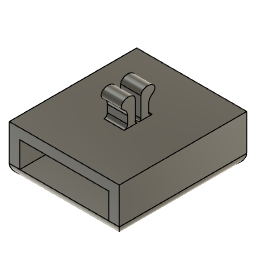
ender5-sd-card-adapter (Autodesk Fusion 360 design; units mm, degrees)
Autodesk Fusion 360 part; units mm, degrees
sketch "Sketch2" plane through (0, 0, 0) normal (0, 0, 1) x (1, 0, 0)
  line L0 (-4.2973, 17.5066) -> (3.1027, 17.5066)
  line L1 (3.1027, 17.5066) -> (3.1027, -15.9934)
  line L2 (3.1027, -15.9934) -> (-4.2973, -15.9934)
  line L3 (-4.2973, -15.9934) -> (-4.2973, 17.5066)
  dimension "d9" = 7.4
  dimension "d10" = 33.5
  constraint horizontal L0
  constraint vertical L1
  constraint horizontal L2
  constraint vertical L3
  measures "d9" distance of L0.start L0.end
  measures "d10" distance of L0.start L2.end
extrude "Extrude1" add sketch "Sketch2" along normal blind 25.5 makes body 1
shell "Shell1" thickness 3 outward yes removed faces 1 at (0.636, -15.9934, 8.5) on bodies 1
sketch "Sketch5" plane through (6.1027, 0, 0) normal (1, 0, 0) x (0, 1, 0)
  line L0 (-15.9934, -3) -> (20.5066, -3)
  line L1 (20.5066, -3) -> (20.5066, 28.5)
  line L2 (20.5066, 28.5) -> (-15.9934, 28.5)
  line L3 (-15.9934, 28.5) -> (-15.9934, -3)
  line L4 (2.2566, 28.5) -> (2.2566, -3) construction
  line L5 (-15.9934, 12.75) -> (20.5066, 12.75) construction
  line L6 (-0.7434, 15.65) -> (1.4566, 15.65)
  line L7 (1.4566, 15.65) -> (1.4566, 9.85)
  line L8 (1.4566, 9.85) -> (-0.7434, 9.85)
  line L9 (-0.7434, 9.85) -> (-0.7434, 15.65)
  line L10 (5.2566, 9.85) -> (5.2566, 15.65)
  line L11 (5.2566, 15.65) -> (3.0566, 15.65)
  line L12 (3.0566, 15.65) -> (3.0566, 9.85)
  line L13 (3.0566, 9.85) -> (5.2566, 9.85)
  dimension "d30" = 5.8
  dimension "d31" = 3
  dimension "d32" = 2.2
  dimension "d33" = 2.9
  constraint midpoint L2 L4.start
  constraint midpoint L0 L4.end
  constraint midpoint L3 L5.start
  constraint midpoint L1 L5.end
  constraint horizontal L6
  constraint vertical L7
  constraint horizontal L8
  constraint vertical L9
  constraint symmetric L4 L6.start L10.end
  constraint symmetric L4 L6.end L11.end
  constraint symmetric L4 L7.end L12.end
  constraint symmetric L4 L8.end L10.start
  measures "d30" distance of L6.start L8.end
  measures "d31" distance of L4 L9
  measures "d32" distance of L6.start L6.end
  measures "d33" distance of L5 L6
extrude "Extrude5" add sketch "Sketch5" along normal blind 6.2 contours L6 L7 L8 L9 | L10 L11 L12 L13 bodies 1
sketch "Sketch7" plane through (0, 0, 15.65) normal (0, 0, 1) x (-1, 0, 0)
  line L0 (-6.1027, -1.4566) -> (-6.1027, 0.7434)
  line L1 (-6.1027, 0.7434) -> (-12.3027, 0.7434)
  line L2 (-12.3027, 0.7434) -> (-12.3027, -1.4566)
  line L3 (-12.3027, -1.4566) -> (-6.1027, -1.4566)
  ellipse E0 centre (-12.3027, 0.5434) end of major axis (-13.8027, 0.5434) minor radius 2
  line L4 (-10.8027, 0.5434) -> (-13.8027, 0.5434)
  line L5 (-12.3027, 2.5434) -> (-12.3027, -1.4566)
  dimension "d41" = 3
  dimension "d42" = 4
  constraint perpendicular L2 L4
  constraint coincident E0 L4.start
  constraint coincident E0 L4.end
  constraint coincident E0 L5.start
  constraint coincident E0 L2.end
  constraint coincident L2.end L3.start
  measures "d41" distance of E0
extrude "Extrude7" add sketch "Sketch7" against normal blind 5.8 contours L2 E0 L4 L5 | L2 E0 L4 L5 | L1 L2 E0 L4 L5 | L1 E0 L5 | L2 E0 L4 L5 bodies 1
fillet "Fillet1" radius 2.25 1 edges at (10.8102, -0.7434, 12.75) on bodies 1
ref_plane "WorkPlane2" through (9.2027, 2.2566, 12.75) normal (0, 1, 0) x (0, 0, 1)
mirror "Mirror2" about plane through (9.2027, 2.2566, 12.75) normal (0, 1, 0) of "Extrude7", "Fillet1"
sketch "Sketch8" plane through (0, 0, 15.65) normal (0, 0, 1) x (-1, 0, 0)
  line L0 (-6.1027, -5.2566) -> (-6.1027, -3.0566)
  line L1 (-6.1027, -3.0566) -> (-12.3027, -3.0566)
  ellipse E0 centre (-12.3027, -5.0566) end of major axis (-12.3027, -3.0566) minor radius 1.5 (-12.3027, -3.0566) -> (-11.1437, -6.3262) ccw
  arc A0 (-9.2282, -5.2566) -> (-11.1437, -6.3262) centre (-9.2282, -7.5066) ccw
  line L2 (-9.2282, -5.2566) -> (-6.1027, -5.2566)
fillet "Fillet2" radius 0.55 2 edges at (6.1027, 3.0566, 12.75) (6.1027, 1.4566, 12.75) on bodies 1
sketch "Sketch1" plane through (0, 0, 0) normal (1, 0, 0) x (0, 1, 0) in component "SDCardThing"
  line L0 (-16.5, -12.5) -> (16.5, -12.5)
  line L1 (16.5, -12.5) -> (16.5, 12.5)
  line L2 (16.5, 12.5) -> (-16.5, 12.5)
  line L3 (-16.5, 12.5) -> (-16.5, -12.5)
  line L4 (-16.5, -12.5) -> (16.5, 12.5) construction
  line L5 (16.5, -12.5) -> (-16.5, 12.5) construction
  dimension "d48" = 33
  dimension "d49" = 25
  constraint horizontal L0
  constraint perpendicular L0 L1
  constraint parallel L0 L2
  constraint parallel L1 L3
  constraint coincident L4 origin
  constraint coincident L5 origin
  measures "d48" distance of L1.end L2.end
  measures "d49" distance of L0.end L1.end
extrude "Extrude1'" add sketch "Sketch1" along normal blind 7.2 separate body makes body 2 in component "SDCardThing"
move_body "Move1" bodies 2 to x (1, 0, 0) y (0, 1, 0) z (0, 0, 1) at (1, 3, 0) in component "SDCardThing"
sketch "Sketch2 (2)" plane through (0, 19.5, 0) normal (0, 1, 0) x (-1, 0, 0) in component "SDCardThing"
  line L0 (-1, -12.5) -> (-1, 12.5)
  line L1 (-1, 12.5) -> (-8.2, 12.5)
  line L2 (-8.2, 12.5) -> (-8.2, -12.5)
  line L3 (-8.2, -12.5) -> (-1, -12.5)
  line L4 (-5.1, -5.5) -> (-4.1, -5.5)
  line L5 (-4.1, -5.5) -> (-4.1, 5.5)
  line L6 (-4.1, 5.5) -> (-5.1, 5.5)
  line L7 (-5.1, 5.5) -> (-5.1, -5.5)
  point P0 (-5.1, 0)
  point P1 (-8.2, 0)
  point P2 (-4.6, -5.5)
  point P3 (-4.6, -12.5)
  dimension "d53" = 1
  dimension "d54" = 11
  constraint horizontal L4
  constraint vertical L5
  constraint horizontal L6
  constraint vertical L7
  constraint midpoint L7 P0
  constraint midpoint L2 P1
  constraint horizontal P0 P1
  constraint midpoint L4 P2
  constraint midpoint L3 P3
  constraint vertical P2 P3
  measures "d53" distance of L4.start L4.end
  measures "d54" distance of L4.start L6.end
extrude "Extrude2" cut sketch "Sketch2 (2)" against normal blind 15 contours L4 L5 L6 L7 bodies 2 in component "SDCardThing"
fillet "Fillet3" radius 1 2 edges at (6.1027, -0.7434, 12.75) (6.1027, 5.2566, 12.75) on bodies 1
sketch "Sketch9" plane through (0, 17.5066, 0) normal (0, -1, 0) x (1, 0, 0)
  line L0 (-4.2973, 0) -> (3.1027, 0)
  line L1 (3.1027, 0) -> (3.1027, 25.5)
  line L2 (3.1027, 25.5) -> (-4.2973, 25.5)
  line L3 (-4.2973, 25.5) -> (-4.2973, 0)
  line L4 (-2.0973, 1.75) -> (0.9027, 1.75)
  line L5 (0.9027, 1.75) -> (0.9027, 23.75)
  line L6 (0.9027, 23.75) -> (-2.0973, 23.75)
  line L7 (-2.0973, 23.75) -> (-2.0973, 1.75)
  line L8 (-4.2973, 0) -> (-4.2973, 25.5)
  point P0 (-2.0973, 12.75)
  point P1 (-4.2973, 12.75)
  dimension "d58" = 3
  dimension "d59" = 22
  dimension "d60" = 2.2
  constraint horizontal L4
  constraint vertical L5
  constraint horizontal L6
  constraint vertical L7
  constraint midpoint L7 P0
  constraint midpoint L8 P1
  constraint horizontal P0 P1
  measures "d58" distance of L4.start L4.end
  measures "d59" distance of L4.start L6.end
  measures "d60" distance of L7 L8
extrude "Extrude8" cut sketch "Sketch9" against normal through all contours L4 L5 L6 L7 bodies 1
sketch "Sketch10" plane through (-7.2973, 0, 0) normal (-1, 0, 0) x (0, -1, 0)
  line L0 (-20.5066, -3) -> (15.9934, -3)
  line L1 (15.9934, -3) -> (15.9934, 28.5)
  line L2 (15.9934, 28.5) -> (-20.5066, 28.5)
  line L3 (-20.5066, 28.5) -> (-20.5066, -3)
  spline S0 degree 3 poles (10.8831, 9.4607) (10.8383, 9.3733) (10.756, 9.2687) (10.7003, 9.2282) knots 0 0 0 0 1 1 1 1
  spline S1 degree 3 poles (10.7003, 9.2282) (10.6017, 9.1565) (10.5631, 9.1616) (9.2299, 9.164) knots 0 0 0 0 1 1 1 1
  line L4 (9.2299, 9.164) -> (2.1139, 9.1771)
  spline S2 degree 3 poles (2.1139, 9.1771) (1.8124, 9.1776) (1.4851, 9.2504) (1.3246, 9.4908) knots 0 0 0 0 1 1 1 1
  line L5 (1.3246, 9.4908) -> (1.2434, 9.6123)
  line L6 (1.2434, 9.6123) -> (0.3224, 12.5525)
  spline S3 degree 3 poles (0.3224, 12.5525) (1.233, 15.3844) (1.2076, 15.3203) (1.4444, 15.3852) knots 0 0 0 0 1 1 1 1
  spline S4 degree 3 poles (1.4444, 15.3852) (1.5355, 15.4448) (1.668, 15.4513) (3.0303, 15.4637) knots 0 0 0 0 1 1 1 1
  line L7 (3.0303, 15.4637) -> (4.5168, 15.4772)
  line L8 (4.5168, 15.4772) -> (5.3578, 16.2918)
  line L9 (5.3578, 16.2918) -> (5.8471, 16.2918)
  line L10 (5.8471, 16.2918) -> (6.3363, 16.2918)
  line L11 (6.3363, 16.2918) -> (6.3363, 16.1142)
  spline S5 degree 3 poles (6.3363, 16.1142) (6.3363, 15.8856) (6.3793, 15.8625) (6.8029, 15.8625) knots 0 0 0 0 1 1 1 1
  line L12 (6.8029, 15.8625) -> (7.1307, 15.8625)
  line L13 (7.1307, 15.8625) -> (7.5578, 16.2688)
  line L14 (7.5578, 16.2688) -> (9.0342, 16.2598)
  spline S6 degree 3 poles (9.0342, 16.2598) (10.3794, 16.2539) (10.5261, 16.2474) (10.6626, 16.1878) knots 0 0 0 0 1 1 1 1
  spline S7 degree 3 poles (10.6626, 16.1878) (10.9617, 16.0567) (10.9418, 16.2902) (10.9549, 12.7529) knots 0 0 0 0 1 1 1 1
  line L15 (10.9549, 12.7529) -> (10.9771, 9.6438)
  line L16 (10.9771, 9.6438) -> (10.8831, 9.4607)
  spline S8 degree 3 poles (5.7859, 15.3324) (5.7789, 15.3326) (5.7718, 15.3326) (5.7645, 15.3324) knots 0 0 0 0 1 1 1 1
  line L17 (8.9549, 14.8454) -> (8.9549, 10.2596)
  line L18 (8.9549, 10.2596) -> (4.989, 12.5525)
  line L19 (4.989, 12.5525) -> (8.9549, 14.8454)
  point P0 (8.9549, 12.5525)
  dimension "d64" = 2
  constraint vertical L17
  constraint horizontal L6.end L18.end
  constraint midpoint L17 P0
  constraint horizontal L18.end P0
  measures "d64" distance of S7.end L17
extrude "Extrude9" cut sketch "Sketch10" against normal blind 1.5 contours S0 S1 L4 S2 L5 L6 S3 S4 L7 L8 L9 L10 L11 S5 L12 L13 L14 S6 S7 L15 L16 bodies 1
fillet "Fillet4" radius 3 4 edges at (-7.2973, 2.2566, 28.5) (-7.2973, 2.2566, -3) (-7.2973, 20.5066, 12.75) (-7.2973, -15.9934, 12.75) on bodies 1
move_body "Move1'" bodies 1 to x (0, 0, 1) y (0, 1, 0) z (-1, 0, 0) at (-10.2973, 0, 4.2973)
move_body "Move2" bodies 2 to x (0, 0, 1) y (0, 1, 0) z (-1, 0, 0) at (-20.2973, 0, -11.7027) in component "SDCardThing"
component "SDCardThing" placed x (1, 0, 0) y (0, 1, 0) z (0, 0, 1) at (-3, 0, 13)
equation "d31 = ( 6 / 2 ) * 1 mm"
equation "d33 = ( 5.8 / 2 ) * 1 mm"
equation "d60 = ( 7.4 / 2 ) * 1 mm - ( ( 3 / 2 ) * 1 mm )"
